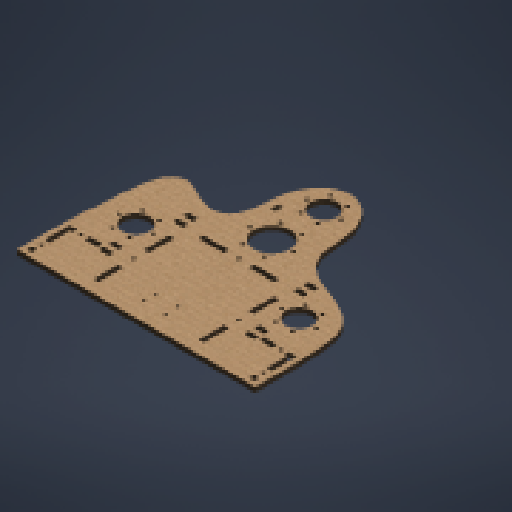
# Autodesk Inventor part: Cart_Floor
Saved by Autodesk Inventor 2024.1 (Build 281209000, 209)
## iProperties
Created: 2023-08-03
Part Number: Cart_Floor
Material: MDF Medium Density Fiberboard
Document SubType Name: Modeling
Designer: jaege
Density: 0.8 g/cm^3
Appearance: Cardboard - Corrugated
Author: jaege
Autodesk Inventor part; units mm, degrees
ref_plane "YZ Plane" through (0, 0, 0) normal (1, 0, 0) x (0, 1, 0)
ref_plane "XZ Plane" through (0, 0, 0) normal (0, 1, 0) x (-1, 0, 0)
ref_plane "XY Plane" through (0, 0, 0) normal (0, 0, 1) x (1, 0, 0)
sketch "Sketch1" plane through (0, 0, 0) normal (0, 1, 0) x (-1, 0, 0)
  line L0 (-40, -40) -> (40, -40) construction
  line L1 (40, -40) -> (40, 40) construction
  line L2 (40, 40) -> (-40, 40) construction
  line L3 (-40, 40) -> (-40, -40) construction
  line L4 (-40, 40) -> (40, 40) construction
  line L5 (40, 40) -> (40, 59.5) construction
  line L6 (40, 59.5) -> (-40, 59.5) construction
  line L7 (-40, 59.5) -> (-40, 40) construction
  circle A0 centre (-65, -24.9396) radius 10.5
  circle A1 centre (0, -68.5) radius 14
  line L8 (-44, 40) -> (44, 40) construction
  line L9 (44, 40) -> (44, -44) construction
  line L10 (44, -44) -> (-44, -44) construction
  line L11 (-44, -44) -> (-44, 40) construction
  line L12 (-100, 59.5) -> (100, 59.5) construction
  line L13 (100, 59.5) -> (100, -140.5) construction
  line L14 (100, -140.5) -> (-100, -140.5) construction
  line L15 (-100, -140.5) -> (-100, 59.5) construction
  line L16 (0, -180.5) -> (0, 99.5) construction
  circle A2 centre (-51.25, -24.9396) radius 1.5
  circle A3 centre (-65, -24.9396) radius 17 construction
  line L17 (-54.5, -24.9396) -> (-48, -24.9396) construction
  circle A4 centre (-58.125, -13.0317) radius 1.5
  circle A5 centre (-71.875, -13.0317) radius 1.5
  circle A6 centre (-78.75, -24.9396) radius 1.5
  circle A7 centre (-71.875, -36.8474) radius 1.5
  circle A8 centre (-58.125, -36.8474) radius 1.5
  circle A9 centre (0, -110) radius 10.5
  circle A10 centre (13.75, -110) radius 1.5
  circle A11 centre (0, -110) radius 17 construction
  line L18 (10.5, -110) -> (17, -110) construction
  circle A12 centre (6.875, -98.0922) radius 1.5
  circle A13 centre (-6.875, -98.0922) radius 1.5
  circle A14 centre (-13.75, -110) radius 1.5
  circle A15 centre (-6.875, -121.9078) radius 1.5
  circle A16 centre (6.875, -121.9078) radius 1.5
  line L19 (-70.6, 27.5) -> (-58.4, 27.5) construction
  line L20 (-58.4, 27.5) -> (-58.4, -4.7) construction
  line L21 (-58.4, -4.7) -> (-70.6, -4.7) construction
  line L22 (-70.6, -4.7) -> (-70.6, 27.5) construction
  circle A17 centre (-64.5, 25.5) radius 1.5
  circle A18 centre (-64.5, -2.7) radius 1.5
  line L23 (-64.5, 27.5) -> (-64.5, -4.7) construction
  line L24 (-70.6, 11.4) -> (-58.4, 11.4) construction
  circle A19 centre (-64.5, 16.5) radius 2.5 construction
  circle A20 centre (17.25, -68.5) radius 1.5
  circle A21 centre (0, -68.5) radius 20.5 construction
  line L25 (14, -68.5) -> (20.5, -68.5) construction
  circle A22 centre (8.625, -53.5611) radius 1.5
  circle A23 centre (-8.625, -53.5611) radius 1.5
  circle A24 centre (-17.25, -68.5) radius 1.5
  circle A25 centre (-8.625, -83.4389) radius 1.5
  circle A26 centre (8.625, -83.4389) radius 1.5
  line L26 (0, 40) -> (-95, 40) construction
  line L27 (-95, 40) -> (-95, 14.5) construction
  line L28 (-95, 14.5) -> (0, 14.5) construction
  line L29 (0, 14.5) -> (0, 40) construction
  line L30 (0, 40) -> (-95, 40) construction
  line L31 (-95, 40) -> (-95, 55.5) construction
  line L32 (-95, 55.5) -> (0, 55.5) construction
  line L33 (0, 55.5) -> (0, 40) construction
  circle A27 centre (-64.5, 16.5) radius 17.5 construction
  line L34 (-44, 14.5) -> (-85, 14.5) construction
  line L35 (-85, 14.5) -> (-85, 55.5) construction
  line L36 (-85, 55.5) -> (-44, 55.5) construction
  line L37 (-44, 55.5) -> (-44, 14.5) construction
  line L38 (-82, 16.5) -> (-82, -24.9396) construction
  circle A28 centre (65, -24.9396) radius 10.5
  circle A29 centre (51.25, -24.9396) radius 1.5
  circle A30 centre (65, -24.9396) radius 17 construction
  line L39 (54.5, -24.9396) -> (48, -24.9396) construction
  circle A31 centre (58.125, -13.0317) radius 1.5
  circle A32 centre (71.875, -13.0317) radius 1.5
  circle A33 centre (78.75, -24.9396) radius 1.5
  circle A34 centre (71.875, -36.8474) radius 1.5
  circle A35 centre (58.125, -36.8474) radius 1.5
  line L40 (70.6, 27.5) -> (58.4, 27.5) construction
  line L41 (58.4, 27.5) -> (58.4, -4.7) construction
  line L42 (58.4, -4.7) -> (70.6, -4.7) construction
  line L43 (70.6, -4.7) -> (70.6, 27.5) construction
  circle A36 centre (64.5, 25.5) radius 1.5
  circle A37 centre (64.5, -2.7) radius 1.5
  line L44 (64.5, 27.5) -> (64.5, -4.7) construction
  line L45 (70.6, 11.4) -> (58.4, 11.4) construction
  circle A38 centre (64.5, 16.5) radius 2.5 construction
  line L46 (0, 40) -> (95, 40) construction
  line L47 (95, 40) -> (95, 14.5) construction
  line L48 (95, 14.5) -> (0, 14.5) construction
  line L49 (0, 40) -> (95, 40) construction
  line L50 (95, 40) -> (95, 55.5) construction
  line L51 (95, 55.5) -> (0, 55.5) construction
  circle A39 centre (64.5, 16.5) radius 17.5 construction
  line L52 (44, 14.5) -> (85, 14.5) construction
  line L53 (85, 14.5) -> (85, 55.5) construction
  line L54 (85, 55.5) -> (44, 55.5) construction
  line L55 (82, 16.5) -> (82, -24.9396) construction
  line L56 (95, 40) -> (-95, 40)
  line L57 (95, 40) -> (95, 14.5)
  line L58 (-95, 40) -> (-95, 14.5)
  spline S0 degree 4 poles (-95, 14.5) (-95, 2.9745) (-92.5859, -15.0646) (-100.8312, -52.3699) (-16.3507, -57.8128) (-37.7982, -109.7894) (0, -145.5519) (37.7982, -109.7894) (16.3507, -57.8128) (100.8312, -52.3699) (92.5859, -15.0646) (95, 2.9745) (95, 14.5) knots 0 0 0 0 0 0.141322 0.242902 0.345989 0.449799 0.550201 0.654011 0.757098 0.858678 1 1 1 1 1
  line L59 (-65, -24.9396) -> (-65, -41.9396) construction
  line L60 (-95, 14.5) -> (-82.6777, -42.6172) construction
  line L61 (-30, -40) -> (-10, -40)
  line L62 (-10, -40) -> (-10, -44)
  line L63 (-10, -44) -> (-30, -44)
  line L64 (-30, -44) -> (-30, -40)
  line L65 (-44, -30) -> (-40, -30)
  line L66 (-40, -30) -> (-40, -10)
  line L67 (-40, -10) -> (-44, -10)
  line L68 (-44, -10) -> (-44, -30)
  line L69 (-44, 30) -> (-40, 30)
  line L70 (-40, 30) -> (-40, 10)
  line L71 (-40, 10) -> (-44, 10)
  line L72 (-44, 10) -> (-44, 30)
  line L73 (30, -40) -> (10, -40)
  line L74 (10, -40) -> (10, -44)
  line L75 (10, -44) -> (30, -44)
  line L76 (30, -44) -> (30, -40)
  line L77 (44, -30) -> (40, -30)
  line L78 (40, -30) -> (40, -10)
  line L79 (40, -10) -> (44, -10)
  line L80 (44, -10) -> (44, -30)
  line L81 (44, 30) -> (40, 30)
  line L82 (40, 30) -> (40, 10)
  line L83 (40, 10) -> (44, 10)
  line L84 (44, 10) -> (44, 30)
  line L85 (-70.6, 22.65) -> (-58.4, 22.65)
  line L86 (-58.4, 22.65) -> (-58.4, 0.15)
  line L87 (-58.4, 0.15) -> (-70.6, 0.15)
  line L88 (-70.6, 0.15) -> (-70.6, 22.65)
  line L89 (70.6, 22.65) -> (58.4, 22.65)
  line L90 (58.4, 22.65) -> (58.4, 0.15)
  line L91 (58.4, 0.15) -> (70.6, 0.15)
  line L92 (70.6, 0.15) -> (70.6, 22.65)
  circle A40 centre (22, 24.5) radius 1.55 construction
  circle A41 centre (10, 19.5) radius 1.55 construction
  circle A42 centre (34, 19.5) radius 1.55 construction
  circle A43 centre (90, 22) radius 1.55 construction
  circle A44 centre (10, 19.5) radius 1.5
  circle A45 centre (22, 24.5) radius 1.5
  circle A46 centre (34, 19.5) radius 1.5
  circle A47 centre (90, 22) radius 1.5
  circle A48 centre (-22, 24.5) radius 1.55 construction
  circle A49 centre (-10, 19.5) radius 1.55 construction
  circle A50 centre (-34, 19.5) radius 1.55 construction
  circle A51 centre (-90, 22) radius 1.55 construction
  circle A52 centre (-10, 19.5) radius 1.5
  circle A53 centre (-22, 24.5) radius 1.5
  circle A54 centre (-34, 19.5) radius 1.5
  circle A55 centre (-90, 22) radius 1.5
  point P0 (0, 0)
  point P1 (0, 59.5)
  point P2 (0, -40)
  point P3 (40, 0)
  point P4 (0, -44)
  point P5 (0, -140.5)
  point P6 (-64.5, 11.4)
  point P7 (-95, 47.75)
  point P8 (-47, 16.5)
  point P9 (-82, 16.5)
  point P10 (0, -48)
  point P11 (0, -89)
  point P12 (0, -93)
  point P13 (64.5, 11.4)
  point P14 (95, 47.75)
  point P15 (47, 16.5)
  point P16 (82, 16.5)
  point P17 (-35, -68.5)
  point P18 (-25, -110)
  point P19 (0, -131)
  point P20 (25, -110)
  point P21 (35, -68.5)
  point P22 (82.6777, -42.6172)
  point P23 (-93.8388, -14.0586)
  point P24 (93.8388, -14.0586)
  point P25 (-88.8388, -14.0586)
  point P26 (-17, -110)
  point P27 (0, -127)
  point P28 (0, -40)
  point P29 (-42, 30)
  point P30 (-58.4, 11.4)
  dimension "d5" = 21
  dimension "d6" = 28
  dimension "d19" = 21
  dimension "d2" = 80
  dimension "d4" = 80
  dimension "d7" = 4
  dimension "d8" = 4
  dimension "d9" = 200
  dimension "d10" = 200
  dimension "d11" = 3
  dimension "d12" = 34
  dimension "d15" = 360
  dimension "d20" = 3
  dimension "d21" = 34
  dimension "d22" = 360
  dimension "d23" = 32.2
  dimension "d24" = 12.2
  dimension "d25" = 3
  dimension "d26" = 5
  dimension "d27" = 9
  dimension "d28" = 28.2
  dimension "d29" = 3
  dimension "d30" = 6.5
  dimension "d33" = 360
  dimension "d36" = 25.5
  dimension "d37" = 41
  dimension "d39" = 95
  dimension "d40" = 35
  dimension "d42" = 4
  dimension "d44" = 39
  dimension "d45" = 3
  dimension "d46" = 21
  dimension "d47" = 3
  dimension "d48" = 3
  dimension "d49" = 4
  dimension "d50" = 4
  dimension "d51" = 25
  dimension "d52" = 45
  dimension "d53" = 5
  dimension "d54" = 35
  dimension "d55" = 8
  dimension "d56" = 4
  dimension "d57" = 20
  dimension "d58" = 20
  dimension "d60" = 10
  dimension "d61" = 10
  dimension "d62" = 20
  dimension "d64" = 10
  dimension "d65" = 22.5
  dimension "d66" = 3
  constraints: 184 end point, 82 horizontal alignment, 48 centre point, 24 parallel, 23 equal radius, 22 coincident, 18 midpoint, 18 point on circle, 15 horizontal, 12 perpendicular, 12 point on line, 8 vertical alignment, 4 vertical, 3 collinear, 2 tangent, 1 symmetric about line, 67 other
  measures "d2" distance of L6.end L5.end
  measures "d4" distance of L0.end L1.end
  measures "d7" distance between parallel lines of L11 L3
  measures "d8" distance between parallel lines of L10 L0
  measures "d9" distance of L12.start L12.end
  measures "d10" distance of L14.end L12.start
  measures "d11" diameter of A2
  measures "d12" diameter of A3
  measures "d20" diameter of A10
  measures "d21" diameter of A11
  measures "d23" distance of L21.end L19.start
  measures "d24" distance of L19.start L19.end
  measures "d25" diameter of A17
  measures "d26" diameter of A19
  measures "d27" distance of A19.centre A17.centre
  measures "d28" distance of A18.centre A17.centre
  measures "d29" diameter of A20
  measures "d36" distance of L26.end L27.end
  measures "d37" distance between parallel lines of L32 L28
  measures "d39" distance of L27.end L28.end
  measures "d40" diameter of A27
  measures "d42" vertical distance of L12.start L31.end
  measures "d44" distance from line of A27.centre L32
  measures "d45" distance from line of L11 A27.start
  measures "d46" distance of L21.end L59.start
  measures "d47" distance from line of A27.end L35
  measures "d48" distance from line of L37 A27.start
  measures "d49" distance of A21.end point (0, -44)
  measures "d50" distance of A11.end point (0, -89)
  measures "d51" distance of L59.start L60.end
  measures "d53" distance of point (-88.839, -14.059) point (-93.839, -14.059)
  measures "d54" distance of point (0, -68.5) point (-35, -68.5)
  measures "d55" distance of point (-17, -110) point (-25, -110)
  measures "d56" distance of point (0, -131) point (0, -127)
  measures "d57" distance of L66.end L65.end
  measures "d58" distance of L69.end L70.end
  measures "d60" distance from line of L0.start L65
  measures "d61" distance of L61.start L0.start
  measures "d62" distance of L61.start L61.end
  measures "d64" distance from line of L26 point (-42, 30)
  measures "d65" distance of L85.end L86.end
  measures "d66" diameter of A44
extrude "Extrusion1" add sketch "Sketch1" along normal blind 4
sketch "Sketch2" plane through (0, 4, 0) normal (0, 1, 0) x (1, 0, 0)
  line L0 (95, -40) -> (95, -14.5) projected
  spline S0 degree 4 poles (95, -14.5) (95, -2.9745) (92.5859, 15.0646) (100.8312, 52.3699) (16.3507, 57.8128) (37.7982, 109.7894) (0, 145.5519) (-37.7982, 109.7894) (-16.3507, 57.8128) (-100.8312, 52.3699) (-92.5859, 15.0646) (-95, -2.9745) (-95, -14.5) knots 0 0 0 0 0 0.141322 0.242902 0.345989 0.449799 0.550201 0.654011 0.757098 0.858678 1 1 1 1 1 projected
  line L1 (-95, -14.5) -> (-95, -40) projected
  line L2 (-95, -40) -> (95, -40) projected
  circle A0 centre (90, -22) radius 1.5 projected
  circle A1 centre (34, -19.5) radius 1.5 projected
  circle A2 centre (10, -19.5) radius 1.5 projected
  circle A3 centre (-90, -22) radius 1.5 projected
  circle A4 centre (-34, -19.5) radius 1.5 projected
  circle A5 centre (-22, -24.5) radius 1.5 projected
  circle A6 centre (-10, -19.5) radius 1.5 projected
  circle A7 centre (-64.5, -25.5) radius 1.5 projected
  circle A8 centre (64.5, -25.5) radius 1.5 projected
  circle A9 centre (22, -24.5) radius 1.5 projected
  line L3 (-70.6, -0.15) -> (-58.4, -0.15) projected
  line L4 (-58.4, -0.15) -> (-58.4, -22.65) projected
  line L5 (-58.4, -22.65) -> (-70.6, -22.65) projected
  line L6 (-70.6, -22.65) -> (-70.6, -0.15) projected
  line L7 (70.6, -22.65) -> (58.4, -22.65) projected
  line L8 (58.4, -22.65) -> (58.4, -0.15) projected
  line L9 (58.4, -0.15) -> (70.6, -0.15) projected
  line L10 (70.6, -0.15) -> (70.6, -22.65) projected
  line L11 (-40, -30) -> (-44, -30) projected
  line L12 (-44, -30) -> (-44, -10) projected
  line L13 (-44, -10) -> (-40, -10) projected
  line L14 (-40, -10) -> (-40, -30) projected
  line L15 (-40, 30) -> (-40, 10) projected
  line L16 (-40, 10) -> (-44, 10) projected
  line L17 (-44, 10) -> (-44, 30) projected
  line L18 (-44, 30) -> (-40, 30) projected
  line L19 (-10, 40) -> (-30, 40) projected
  line L20 (-30, 40) -> (-30, 44) projected
  line L21 (-30, 44) -> (-10, 44) projected
  line L22 (-10, 44) -> (-10, 40) projected
  line L23 (44, -30) -> (40, -30) projected
  line L24 (40, -30) -> (40, -10) projected
  line L25 (40, -10) -> (44, -10) projected
  line L26 (44, -10) -> (44, -30) projected
  line L27 (44, 30) -> (44, 10) projected
  line L28 (44, 10) -> (40, 10) projected
  line L29 (40, 10) -> (40, 30) projected
  line L30 (40, 30) -> (44, 30) projected
  line L31 (30, 40) -> (10, 40) projected
  line L32 (10, 40) -> (10, 44) projected
  line L33 (10, 44) -> (30, 44) projected
  line L34 (30, 44) -> (30, 40) projected
  circle A10 centre (-78.75, 24.9396) radius 1.5 projected
  circle A11 centre (-64.5, 2.7) radius 1.5 projected
  circle A12 centre (-58.125, 36.8474) radius 1.5 projected
  circle A13 centre (-71.875, 36.8474) radius 1.5 projected
  circle A14 centre (-71.875, 13.0317) radius 1.5 projected
  circle A15 centre (-58.125, 13.0317) radius 1.5 projected
  circle A16 centre (-51.25, 24.9396) radius 1.5 projected
  circle A17 centre (-65, 24.9396) radius 10.5 projected
  circle A18 centre (-8.625, 83.4389) radius 1.5 projected
  circle A19 centre (8.625, 83.4389) radius 1.5 projected
  circle A20 centre (17.25, 68.5) radius 1.5 projected
  circle A21 centre (8.625, 53.5611) radius 1.5 projected
  circle A22 centre (-8.625, 53.5611) radius 1.5 projected
  circle A23 centre (-17.25, 68.5) radius 1.5 projected
  circle A24 centre (64.5, 2.7) radius 1.5 projected
  circle A25 centre (6.875, 98.0922) radius 1.5 projected
  circle A26 centre (13.75, 110) radius 1.5 projected
  circle A27 centre (0, 110) radius 10.5 projected
  circle A28 centre (-6.875, 121.9078) radius 1.5 projected
  circle A29 centre (6.875, 121.9078) radius 1.5 projected
  circle A30 centre (-6.875, 98.0922) radius 1.5 projected
  circle A31 centre (-13.75, 110) radius 1.5 projected
  circle A32 centre (58.125, 36.8474) radius 1.5 projected
  circle A33 centre (71.875, 36.8474) radius 1.5 projected
  circle A34 centre (78.75, 24.9396) radius 1.5 projected
  circle A35 centre (71.875, 13.0317) radius 1.5 projected
  circle A36 centre (58.125, 13.0317) radius 1.5 projected
  circle A37 centre (51.25, 24.9396) radius 1.5 projected
  circle A38 centre (0, 68.5) radius 14 projected
  circle A39 centre (65, 24.9396) radius 10.5 projected
  point P0 (0, 0)
  constraints: 1 horizontal alignment
extrude "Extrusion2" add sketch "Sketch2" against normal up to surface (4 mm away) contours L2 L1 S0 L0 | A0 | A1 | A2 | A3 | A4 | A5 | A6 | A7 | A8 | A9 | L3 L4 L5 L6 | L7 L8 L9 L10 | A11 | A24
sketch "Sketch3" plane through (0, 4, 0) normal (0, 1, 0) x (1, 0, 0)
  line L0 (-54, -7.845) -> (-62, -7.845)
  line L1 (-62, -7.845) -> (-62, -3.845)
  line L2 (-62, -3.845) -> (-54, -3.845)
  line L3 (-54, -3.845) -> (-54, -7.845)
  line L4 (-54, 0.155) -> (-62, 0.155)
  line L5 (-62, 0.155) -> (-62, 4.155)
  line L6 (-62, 4.155) -> (-54, 4.155)
  line L7 (-54, 4.155) -> (-54, 0.155)
  arc A0 (-65, 7.9396) -> (-65, 41.9396) centre (-65, 24.9396) ccw construction
  line L8 (-44, -30) -> (-44, -10) projected
  line L9 (-44, 41.432) -> (-52, 41.432)
  line L10 (-52, 41.432) -> (-52, 45.432)
  line L11 (-52, 45.432) -> (-44, 45.432)
  line L12 (-44, 45.432) -> (-44, 41.432)
  line L13 (-44, 49.432) -> (-52, 49.432)
  line L14 (-52, 49.432) -> (-52, 53.432)
  line L15 (-52, 53.432) -> (-44, 53.432)
  line L16 (-44, 53.432) -> (-44, 49.432)
  line L17 (-30, 40) -> (-30, 44) projected
  line L18 (0, 0) -> (0, 131) construction
  line L19 (54, -7.845) -> (62, -7.845)
  line L20 (62, -7.845) -> (62, -3.845)
  line L21 (62, -3.845) -> (54, -3.845)
  line L22 (54, -3.845) -> (54, -7.845)
  line L23 (54, 0.155) -> (62, 0.155)
  line L24 (62, 0.155) -> (62, 4.155)
  line L25 (62, 4.155) -> (54, 4.155)
  line L26 (54, 4.155) -> (54, 0.155)
  arc A1 (65, 41.9396) -> (65, 7.9396) centre (65, 24.9396) ccw construction
  line L27 (44, 41.432) -> (52, 41.432)
  line L28 (52, 41.432) -> (52, 45.432)
  line L29 (52, 45.432) -> (44, 45.432)
  line L30 (44, 45.432) -> (44, 41.432)
  line L31 (44, 49.432) -> (52, 49.432)
  line L32 (52, 49.432) -> (52, 53.432)
  line L33 (52, 53.432) -> (44, 53.432)
  line L34 (44, 53.432) -> (44, 49.432)
  point P0 (44, -10)
  point P1 (-44, 30)
  dimension "d69" = 8
  dimension "d70" = 4
  dimension "d71" = 8
  dimension "d72" = 4
  dimension "d73" = 4
  dimension "d74" = 21
  dimension "d75" = 10
  dimension "d76" = 8
  dimension "d77" = 4
  dimension "d78" = 8
  dimension "d79" = 4
  dimension "d80" = 4
  dimension "d81" = 21
  constraints: 66 end point, 20 symmetric about line, 8 parallel, 4 horizontal, 4 perpendicular, 4 point on circle, 4 point on line, 2 centre point, 1 vertical, 1 vertical alignment, 7 other
  measures "d69" distance of L1.end L2.end
  measures "d70" distance of L0.end L1.end
  measures "d71" distance of L5.end L6.end
  measures "d72" distance of L4.end L5.end
  measures "d73" distance of L1.end L4.end
  measures "d74" distance of L5.end A0.centre
  measures "d75" distance from line of L8 L0.start
  measures "d76" distance of L10.end L11.end
  measures "d77" distance of L9.end L10.end
  measures "d78" distance of L14.end L15.end
  measures "d79" distance of L13.end L14.end
  measures "d80" distance of L10.end L13.end
  measures "d81" distance of A0.centre L9.end
extrude "Extrusion3" cut sketch "Sketch3" against normal blind 10
sketch "Sketch4" plane through (0, 4, 0) normal (0, 1, 0) x (1, 0, 0)
  line L0 (-21.9772, 95.1455) -> (-17.9772, 95.1455)
  line L1 (-17.9772, 95.1455) -> (-17.9772, 89.1455)
  line L2 (-17.9772, 89.1455) -> (-21.9772, 89.1455)
  line L3 (-21.9772, 89.1455) -> (-21.9772, 95.1455)
  line L4 (-21.9772, 95.1455) -> (-17.9772, 95.1455)
  line L5 (-17.9772, 95.1455) -> (-17.9772, 99.1455) construction
  line L6 (-17.9772, 99.1455) -> (-21.9772, 99.1455) construction
  line L7 (-21.9772, 99.1455) -> (-21.9772, 95.1455) construction
  line L8 (-21.9772, 89.1455) -> (-17.9772, 89.1455)
  line L9 (-17.9772, 89.1455) -> (-17.9772, 85.1455) construction
  line L10 (-17.9772, 85.1455) -> (-21.9772, 85.1455) construction
  line L11 (-21.9772, 85.1455) -> (-21.9772, 89.1455) construction
  arc A0 (0, 127) -> (0, 93) centre (0, 110) ccw
  arc A1 (0, 89) -> (0, 48) centre (0, 68.5) ccw
  point P0 (0, 0)
  dimension "d85" = 4
  dimension "d86" = 6
  dimension "d87" = 4
  dimension "d88" = 4
  dimension "d89" = 4
  dimension "d90" = 4
  dimension "d91" = 21
  dimension "d92" = 24.5
  constraints: 24 end point, 6 parallel, 4 point on circle, 3 horizontal, 3 perpendicular, 2 centre point, 8 other
  measures "d85" distance of L1.end L2.end
  measures "d86" distance of L0.end L1.end
  measures "d87" distance of L6.end L5.end
  measures "d88" distance of L5.end L4.end
  measures "d89" distance of L9.end L10.end
  measures "d90" distance of L8.end L9.end
  measures "d91" distance of A0.centre L5.end
  measures "d92" distance of L9.end A1.centre
extrude "Extrusion4" cut sketch "Sketch4" against normal up to surface (4 mm away)
sketch "Sketch5" plane through (0, 4, 0) normal (0, 1, 0) x (1, 0, 0)
  spline S0 degree 4 poles (95, -14.5) (95, -2.9745) (92.5859, 15.0646) (100.8312, 52.3699) (16.3507, 57.8128) (37.7982, 109.7894) (0, 145.5519) (-37.7982, 109.7894) (-16.3507, 57.8128) (-100.8312, 52.3699) (-92.5859, 15.0646) (-95, -2.9745) (-95, -14.5) knots 0 0 0 0 0 0.141322 0.242902 0.345989 0.449799 0.550201 0.654011 0.757098 0.858678 1 1 1 1 1
  spline S1 degree 4 poles (-93.2021, 20.5) (-91.4106, 34.039) (-94.091, 75.758) (-73.3181, 80.9043) (-53.2896, 63.1758) (-31.666, 63.6765) (-29.5431, 78.4083) (-28.7201, 85.5) knots 0 0 0 0 0 0.388489 0.569164 0.715257 1 1 1 1 1
  line L0 (-94.3927, 11.5024) -> (-92.0115, 29.4976) construction
  arc A0 (-94.7142, 13.4703) -> (-92.8338, 27.6811) centre (-137.6289, 26.3788) ccw construction
  line L1 (-54.076, 65.5) -> (-35.924, 65.5) construction
  arc A1 (-51.8339, 66.6893) -> (-38.1661, 66.6893) centre (-45, 85.7283) ccw construction
  line L2 (-80.4456, 75.5) -> (-69.5544, 75.5) construction
  arc A2 (-70.8614, 74.8372) -> (-79.1386, 74.8372) centre (-75, 62.2479) ccw construction
  point P0 (0, 0)
  point P1 (-75, 75.5)
  point P2 (-45, 65.5)
  point P3 (-32.7756, 71.6543)
  dimension "d95" = 35
  dimension "d96" = 100
  dimension "d97" = 80
  dimension "d98" = 90
  dimension "d99" = 20
  dimension "d100" = 50
  dimension "d101" = 0.6
  dimension "d102" = 1
  dimension "d103" = 1
  constraints: 6 end point, 6 midpoint, 4 horizontal, 3 centre point, 3 point on circle, 15 other
  measures "d95" vertical distance of point (-95, -14.5) point (-93.202, 20.5)
  measures "d96" vertical distance of point (-95, -14.5) point (-28.72, 85.5)
  measures "d97" vertical distance of point (-95, -14.5) point (-45, 65.5)
  measures "d98" vertical distance of point (-95, -14.5) point (-75, 75.5)
  measures "d99" horizontal distance of point (-75, 75.5) point (-95, -14.5)
  measures "d100" horizontal distance of point (-45, 65.5) point (-95, -14.5)
extrude "Extrusion5" add sketch "Sketch5" against normal up to surface (4 mm away) contours S0 S1 picked at (-76.8057, 64.3705)
sketch "Sketch6" plane through (0, 0, 0) normal (0, -1, 0) x (1, 0, 0)
  circle A0 centre (-8.9, 24.85) radius 1.175
  circle A1 centre (-8.9, 15.35) radius 1.175
  circle A2 centre (8.9, 15.35) radius 1.175
  circle A3 centre (8.9, 24.85) radius 1.175
  line L0 (-40, 10) -> (-40, 30) construction
  line L1 (40, 30) -> (40, 10) construction
  line L2 (-95, 40) -> (95, 40) projected
  point P0 (0, 0)
  dimension "d106" = 31.1
  dimension "d107" = 2.35
  dimension "d108" = 15.15
  dimension "d109" = 9.5
  dimension "d110" = 31.1
  constraints: 4 centre point, 3 equal radius, 2 horizontal alignment, 2 vertical alignment
  measures "d106" distance from line of L1 A3.centre
  measures "d107" diameter of A3
  measures "d108" distance from line of L2 A3.centre
  measures "d109" distance of A2.centre A3.centre
  measures "d110" distance from line of L0 A0.centre
extrude "Extrusion6" cut sketch "Sketch6" against normal up to next
sketch "Sketch7" plane through (0, 0, 0) normal (0, -1, 0) x (1, 0, 0)
  line L0 (-40, 10) -> (-40, 30) construction
  line L1 (-95, 40) -> (95, 40) construction
  line L2 (-64.6, 6.2) -> (-74.6, 6.2)
  line L3 (-74.6, 6.2) -> (-74.6, 2.2)
  line L4 (-74.6, 2.2) -> (-64.6, 2.2)
  line L5 (-64.6, 2.2) -> (-64.6, 6.2)
  line L6 (-84.6, 2.2) -> (-90.6, 2.2)
  line L7 (-90.6, 2.2) -> (-90.6, 6.2)
  line L8 (-90.6, 6.2) -> (-84.6, 6.2)
  line L9 (-84.6, 6.2) -> (-84.6, 2.2)
  circle A0 centre (-79.6, 4.2) radius 1.5
  line L10 (-74.6, 4.2) -> (-79.6, 4.2) construction
  line L11 (-79.6, 4.2) -> (-84.6, 4.2) construction
  line L12 (-64.6, 10.2) -> (-74, 10.2) construction
  line L13 (-74, 10.2) -> (-74, 30) construction
  line L14 (-74, 30) -> (-64.6, 30) construction
  line L15 (-64.6, 30) -> (-64.6, 10.2) construction
  line L16 (-95, 40) -> (95, 40) projected
  line L17 (-90.6, 6.2) -> (-86.6, 6.2)
  line L18 (-86.6, 6.2) -> (-86.6, 22.2)
  line L19 (-86.6, 22.2) -> (-90.6, 22.2)
  line L20 (-90.6, 22.2) -> (-90.6, 6.2)
  line L21 (-90.6, 32.2) -> (-86.6, 32.2)
  line L22 (-86.6, 32.2) -> (-86.6, 36.2)
  line L23 (-86.6, 36.2) -> (-90.6, 36.2)
  line L24 (-90.6, 36.2) -> (-90.6, 32.2)
  circle A1 centre (-88.6, 27.2) radius 1.5
  line L25 (-88.6, 32.2) -> (-88.6, 27.2) construction
  line L26 (-88.6, 27.2) -> (-88.6, 22.2) construction
  line L27 (0, 40) -> (0, 0) construction
  line L28 (64.6, 6.2) -> (74.6, 6.2)
  line L29 (74.6, 6.2) -> (74.6, 2.2)
  line L30 (74.6, 2.2) -> (64.6, 2.2)
  line L31 (64.6, 2.2) -> (64.6, 6.2)
  line L32 (84.6, 2.2) -> (90.6, 2.2)
  line L33 (90.6, 2.2) -> (90.6, 6.2)
  line L34 (90.6, 6.2) -> (84.6, 6.2)
  line L35 (84.6, 6.2) -> (84.6, 2.2)
  circle A2 centre (79.6, 4.2) radius 1.5
  line L36 (74.6, 4.2) -> (79.6, 4.2) construction
  line L37 (79.6, 4.2) -> (84.6, 4.2) construction
  line L38 (64.6, 10.2) -> (74, 10.2) construction
  line L39 (74, 10.2) -> (74, 30) construction
  line L40 (74, 30) -> (64.6, 30) construction
  line L41 (64.6, 30) -> (64.6, 10.2) construction
  line L42 (90.6, 6.2) -> (86.6, 6.2)
  line L43 (86.6, 6.2) -> (86.6, 22.2)
  line L44 (86.6, 22.2) -> (90.6, 22.2)
  line L45 (90.6, 22.2) -> (90.6, 6.2)
  line L46 (90.6, 32.2) -> (86.6, 32.2)
  line L47 (86.6, 32.2) -> (86.6, 36.2)
  line L48 (86.6, 36.2) -> (90.6, 36.2)
  line L49 (90.6, 36.2) -> (90.6, 32.2)
  circle A3 centre (88.6, 27.2) radius 1.5
  line L50 (88.6, 32.2) -> (88.6, 27.2) construction
  line L51 (88.6, 27.2) -> (88.6, 22.2) construction
  point P0 (-60, 22.25)
  point P1 (60, 22.25)
  dimension "d113" = 20
  dimension "d114" = 17.75
  dimension "d115" = 10
  dimension "d116" = 4
  dimension "d117" = 6
  dimension "d118" = 10
  dimension "d119" = 3
  dimension "d120" = 9.4
  dimension "d121" = 19.8
  dimension "d122" = 4.6
  dimension "d123" = 4
  dimension "d124" = 10
  dimension "d125" = 4
  dimension "d126" = 4
  dimension "d127" = 10
  dimension "d129" = 16
  dimension "d130" = 3
  constraints: 98 end point, 27 symmetric about line, 11 equal length, 6 horizontal, 6 point on line, 5 midpoint, 5 perpendicular, 4 centre point, 4 vertical alignment, 2 coincident, 2 collinear, 1 horizontal alignment, 1 vertical, 2 other
  measures "d113" distance from line of L0 point (-60, 22.25)
  measures "d114" distance from line of L1 point (-60, 22.25)
  measures "d115" distance of L4.end L3.end
  measures "d116" distance of L3.end L2.end
  measures "d117" distance of L7.end L8.end
  measures "d118" distance from line of L10.start L9
  measures "d119" diameter of A0
  measures "d120" distance of L13.end L14.end
  measures "d121" distance of L12.end L13.end
  measures "d122" distance from line of L15 point (-60, 22.25)
  measures "d123" distance between parallel lines of L2 L12
  measures "d124" distance between parallel lines of L14 L16
  measures "d125" distance of L22.end L23.end
  measures "d126" distance of L23.end L21.start
  measures "d127" distance between parallel lines of L19 L21
  measures "d129" distance of L19.end L17.start
  measures "d130" diameter of A1
extrude "Extrusion7" cut sketch "Sketch7" against normal up to next
sketch "Sketch8" plane through (0, 0, 0) normal (0, -1, 0) x (1, 0, 0)
  circle A0 centre (79.6, 4.2) radius 1.5 construction
  line L0 (-84.6, 2.2) -> (-90.6, 2.2) construction
  line L1 (-90.6, 2.2) -> (-90.6, 22.2) construction
  line L2 (-90.6, 22.2) -> (-86.6, 22.2) construction
  line L3 (-86.6, 22.2) -> (-86.6, 6.2) construction
  line L4 (-86.6, 6.2) -> (-84.6, 6.2) construction
  line L5 (-84.6, 6.2) -> (-84.6, 2.2) construction
  line L6 (-64.6, 2.2) -> (-74.6, 2.2) construction
  line L7 (-74.6, 2.2) -> (-74.6, 6.2) construction
  line L8 (-74.6, 6.2) -> (-64.6, 6.2) construction
  line L9 (-64.6, 6.2) -> (-64.6, 2.2) construction
  line L10 (-90.6, 36.2) -> (-86.6, 36.2) construction
  line L11 (-86.6, 36.2) -> (-86.6, 32.2) construction
  line L12 (-86.6, 32.2) -> (-90.6, 32.2) construction
  line L13 (-90.6, 32.2) -> (-90.6, 36.2) construction
  line L14 (86.6, 6.2) -> (86.6, 22.2) construction
  line L15 (86.6, 22.2) -> (90.6, 22.2) construction
  line L16 (90.6, 22.2) -> (90.6, 2.2) construction
  line L17 (90.6, 2.2) -> (84.6, 2.2) construction
  line L18 (84.6, 2.2) -> (84.6, 6.2) construction
  line L19 (84.6, 6.2) -> (86.6, 6.2) construction
  circle A1 centre (88.6, 27.2) radius 1.5 construction
  circle A2 centre (-88.6, 27.2) radius 1.5 construction
  circle A3 centre (-79.6, 4.2) radius 1.5 construction
  line L20 (74.6, 2.2) -> (64.6, 2.2) construction
  line L21 (64.6, 2.2) -> (64.6, 6.2) construction
  line L22 (64.6, 6.2) -> (74.6, 6.2) construction
  line L23 (74.6, 6.2) -> (74.6, 2.2) construction
  line L24 (86.6, 32.2) -> (86.6, 36.2) construction
  line L25 (86.6, 36.2) -> (90.6, 36.2) construction
  line L26 (90.6, 36.2) -> (90.6, 32.2) construction
  line L27 (90.6, 32.2) -> (86.6, 32.2) construction
  circle A4 centre (-8.9, 15.35) radius 1.175 construction
  circle A5 centre (8.9, 15.35) radius 1.175 construction
  circle A6 centre (8.9, 24.85) radius 1.175 construction
  circle A7 centre (-8.9, 24.85) radius 1.175 construction
  line L28 (-17.9772, -95.1455) -> (-21.9772, -95.1455) construction
  line L29 (-21.9772, -95.1455) -> (-21.9772, -89.1455) construction
  line L30 (-21.9772, -89.1455) -> (-17.9772, -89.1455) construction
  line L31 (-17.9772, -89.1455) -> (-17.9772, -95.1455) construction
  line L32 (52, -53.432) -> (44, -53.432) construction
  line L33 (44, -53.432) -> (44, -49.432) construction
  line L34 (44, -49.432) -> (52, -49.432) construction
  line L35 (52, -49.432) -> (52, -53.432) construction
  line L36 (-62, -4.155) -> (-62, -0.155) construction
  line L37 (-62, -0.155) -> (-54, -0.155) construction
  line L38 (-54, -0.155) -> (-54, -4.155) construction
  line L39 (-54, -4.155) -> (-62, -4.155) construction
  line L40 (-52, -45.432) -> (-52, -41.432) construction
  line L41 (-52, -41.432) -> (-44, -41.432) construction
  line L42 (-44, -41.432) -> (-44, -45.432) construction
  line L43 (-44, -45.432) -> (-52, -45.432) construction
  line L44 (62, -0.155) -> (62, -4.155) construction
  line L45 (62, -4.155) -> (54, -4.155) construction
  line L46 (54, -4.155) -> (54, -0.155) construction
  line L47 (54, -0.155) -> (62, -0.155) construction
  line L48 (44, -45.432) -> (44, -41.432) construction
  line L49 (44, -41.432) -> (52, -41.432) construction
  line L50 (52, -41.432) -> (52, -45.432) construction
  line L51 (52, -45.432) -> (44, -45.432) construction
  line L52 (-62, 3.845) -> (-62, 7.845) construction
  line L53 (-62, 7.845) -> (-54, 7.845) construction
  line L54 (-54, 7.845) -> (-54, 3.845) construction
  line L55 (-54, 3.845) -> (-62, 3.845) construction
  line L56 (-52, -53.432) -> (-52, -49.432) construction
  line L57 (-52, -49.432) -> (-44, -49.432) construction
  line L58 (-44, -49.432) -> (-44, -53.432) construction
  line L59 (-44, -53.432) -> (-52, -53.432) construction
  line L60 (62, 3.845) -> (54, 3.845) construction
  line L61 (54, 3.845) -> (54, 7.845) construction
  line L62 (54, 7.845) -> (62, 7.845) construction
  line L63 (62, 7.845) -> (62, 3.845) construction
  line L64 (95, 40) -> (95, 14.5) construction
  line L65 (-95, 40) -> (95, 40) construction
  line L66 (-95, 14.5) -> (-95, 40) construction
  line L67 (-40, 30) -> (-44, 30) construction
  line L68 (-40, 10) -> (-40, 30) construction
  line L69 (-44, 10) -> (-40, 10) construction
  line L70 (-44, 30) -> (-44, 10) construction
  line L71 (-40, -30) -> (-40, -10) construction
  line L72 (-44, -30) -> (-40, -30) construction
  line L73 (-44, -10) -> (-44, -30) construction
  line L74 (-40, -10) -> (-44, -10) construction
  line L75 (-10, -40) -> (-30, -40) construction
  line L76 (-10, -44) -> (-10, -40) construction
  line L77 (-30, -44) -> (-10, -44) construction
  line L78 (-30, -40) -> (-30, -44) construction
  line L79 (44, 30) -> (40, 30) construction
  line L80 (44, 10) -> (44, 30) construction
  line L81 (40, 10) -> (44, 10) construction
  line L82 (40, 30) -> (40, 10) construction
  line L83 (44, -30) -> (44, -10) construction
  line L84 (40, -30) -> (44, -30) construction
  line L85 (40, -10) -> (40, -30) construction
  line L86 (44, -10) -> (40, -10) construction
  line L87 (30, -40) -> (10, -40) construction
  line L88 (30, -44) -> (30, -40) construction
  line L89 (10, -44) -> (30, -44) construction
  line L90 (10, -40) -> (10, -44) construction
  circle A8 centre (-78.75, -24.9396) radius 1.5 construction
  circle A9 centre (-58.125, -36.8474) radius 1.5 construction
  circle A10 centre (-71.875, -36.8474) radius 1.5 construction
  circle A11 centre (-71.875, -13.0317) radius 1.5 construction
  circle A12 centre (-58.125, -13.0317) radius 1.5 construction
  circle A13 centre (-51.25, -24.9396) radius 1.5 construction
  circle A14 centre (-65, -24.9396) radius 10.5 construction
  circle A15 centre (-8.625, -83.4389) radius 1.5 construction
  circle A16 centre (8.625, -83.4389) radius 1.5 construction
  circle A17 centre (17.25, -68.5) radius 1.5 construction
  circle A18 centre (8.625, -53.5611) radius 1.5 construction
  circle A19 centre (-8.625, -53.5611) radius 1.5 construction
  circle A20 centre (-17.25, -68.5) radius 1.5 construction
  circle A21 centre (6.875, -98.0922) radius 1.5 construction
  circle A22 centre (13.75, -110) radius 1.5 construction
  circle A23 centre (0, -110) radius 10.5 construction
  circle A24 centre (-6.875, -121.9078) radius 1.5 construction
  circle A25 centre (6.875, -121.9078) radius 1.5 construction
  circle A26 centre (-6.875, -98.0922) radius 1.5 construction
  circle A27 centre (-13.75, -110) radius 1.5 construction
  circle A28 centre (58.125, -36.8474) radius 1.5 construction
  circle A29 centre (71.875, -36.8474) radius 1.5 construction
  circle A30 centre (78.75, -24.9396) radius 1.5 construction
  circle A31 centre (71.875, -13.0317) radius 1.5 construction
  circle A32 centre (58.125, -13.0317) radius 1.5 construction
  circle A33 centre (51.25, -24.9396) radius 1.5 construction
  circle A34 centre (0, -68.5) radius 14 construction
  circle A35 centre (65, -24.9396) radius 10.5 construction
  line L91 (-44, 10) -> (-40, -10) construction
  line L92 (-10, -44) -> (10, -40) construction
  line L93 (40, -10) -> (44, 10) construction
  circle A36 centre (-42, 0) radius 1.5
  circle A37 centre (0, -42) radius 1.5
  circle A38 centre (42, 0) radius 1.5
  point P0 (0, 0)
  dimension "d133" = 3
  constraints: 6 end point, 3 centre point, 3 midpoint, 2 equal radius, 1 perpendicular, 3 other
  measures "d133" diameter of A36
extrude "Extrusion8" cut sketch "Sketch8" against normal up to next
body "Solid1"
